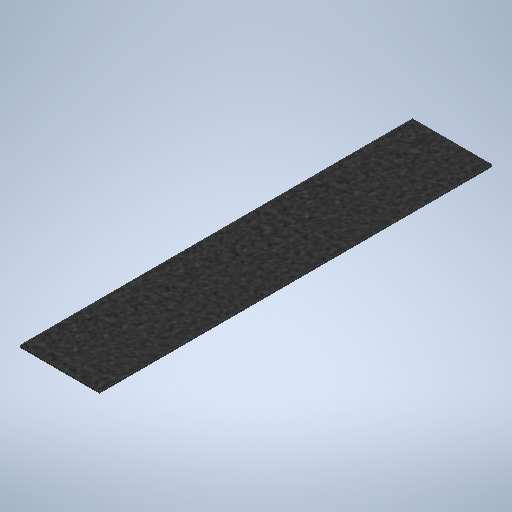
# Autodesk Inventor part: Starter_Shingle_With_Dimensions_6.5_x_30.389_Inches
Saved by Autodesk Inventor 2025.1 (Build 291241020, 241B)
## iProperties
Created: 2024-10-02
Part Number: Starter_Shingle_With_Dimensions_6.5_x_30.389_Inches
Material: Generic
Document SubType Name: Modeling
Designer: Tom
Density: 1 g/cm^3
Appearance: Asphalt 2
Author: Tom
Autodesk Inventor part; units mm, degrees
ref_plane "YZ Plane" through (0, 0, 0) normal (1, 0, 0) x (0, 1, 0)
ref_plane "XZ Plane" through (0, 0, 0) normal (0, 1, 0) x (-1, 0, 0)
ref_plane "XY Plane" through (0, 0, 0) normal (0, 0, 1) x (1, 0, 0)
sketch "Sketch1" plane through (0, 0, 0) normal (0, 1, 0) x (-1, 0, 0)
  line L0 (0, 0) -> (165.1, 0)
  line L1 (165.1, 0) -> (165.1, -814.705)
  line L2 (165.1, -814.705) -> (0, -814.705)
  line L3 (0, -814.705) -> (0, 0)
  dimension "d0" = 165.1
  dimension "d1" = 814.705
  constraints: 8 end point, 2 parallel, 1 horizontal, 1 perpendicular
  measures "d0" distance of L0.start L0.end
  measures "d1" distance of L2.end L0.start
extrude "Extrusion1" add sketch "Sketch1" along normal blind 3.175
body "Solid1"
